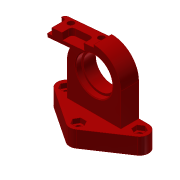
# Autodesk Inventor part: CyclmarcoTraseroY
Saved by Autodesk Inventor 2015 SP2 (Build 190223200, 223)
## iProperties
Created: 2015-05-19
Material: Genérico
Document SubType Name: Modeling
Designer: E.Beroiz
Density: 1 g/cm^3
Appearance: Suave - Rojo
Description: CyclmarcoTraseroY
Author: EDU
Autodesk Inventor part; units mm, degrees
sketch "Boceto1" plane through (0, 0, 0) normal (0, 0, 1) x (1, 0, 0)
  line L0 (-3.0509, -4.5763) -> (-25.5509, 10.4237)
  arc A0 (-22.5, 20.5) -> (-25.5509, 10.4237) centre (-22.5, 15) ccw
  line L1 (-22.5, 20.5) -> (22.5, 20.5)
  arc A1 (25.5509, 10.4237) -> (22.5, 20.5) centre (22.5, 15) ccw
  line L2 (25.5509, 10.4237) -> (3.0509, -4.5763)
  arc A2 (-3.0509, -4.5763) -> (3.0509, -4.5763) centre (0, 0) ccw
  line L3 (22.5, 15) -> (-22.5, 15) construction
  line L4 (0, 15) -> (0, 0) construction
  dimension "d0" = 45
  dimension "d1" = 5.5
  dimension "d2" = 5.5
  dimension "d3" = 5.5
  dimension "d98" = 15
  constraints: 10 end point, 6 point on circle, 6 tangent, 3 centre point, 3 coincident, 1 horizontal, 1 midpoint, 1 perpendicular
  measures "d0" distance of L3.end L3.start
  measures "d1" radius of A1
  measures "d2" radius of A2
  measures "d3" radius of A0
  measures "d98" distance of L4.start L4.end
extrude "Extrusión1" add sketch "Boceto1" along normal blind 10
hole "Agujero1" at (-22.5, 15, 10) direction (0, 0, -1) diameter 3.75 end through all
hole "Agujero2" at (0, 0, 10) direction (0, 0, -1) diameter 3.75 end through all
hole "Agujero3" at (22.5, 15, 10) direction (0, 0, -1) diameter 3.75 end through all
sketch "Boceto3" plane through (0, 0, 10) normal (0, 0, 1) x (1, 0, 0)
  circle A0 centre (22.5, 15) radius 1.875 projected
  circle A1 centre (0, 0) radius 1.875 projected
  circle A2 centre (-22.5, 15) radius 1.875 projected
  line L0 (-25.5509, 10.4237) -> (-3.0509, -4.5763) projected
  arc A3 (-3.0509, -4.5763) -> (3.0509, -4.5763) centre (0, 0) ccw projected
  line L1 (3.0509, -4.5763) -> (25.5509, 10.4237) projected
  arc A4 (25.5509, 10.4237) -> (22.5, 20.5) centre (22.5, 15) ccw projected
  line L2 (22.5, 20.5) -> (-22.5, 20.5) projected
  arc A5 (-22.5, 20.5) -> (-25.5509, 10.4237) centre (-22.5, 15) ccw projected
  line L3 (-20.7001, 18.1175) -> (-18.9002, 15)
  line L4 (-18.9002, 15) -> (-20.7001, 11.8825)
  line L5 (-20.7001, 11.8825) -> (-24.2999, 11.8825)
  line L6 (-24.2999, 11.8825) -> (-26.0998, 15)
  line L7 (-26.0998, 15) -> (-24.2999, 18.1175)
  line L8 (-24.2999, 18.1175) -> (-20.7001, 18.1175)
  line L9 (1.7999, 3.1175) -> (3.5998, 0)
  line L10 (3.5998, 0) -> (1.7999, -3.1175)
  line L11 (1.7999, -3.1175) -> (-1.7999, -3.1175)
  line L12 (-1.7999, -3.1175) -> (-3.5998, 0)
  line L13 (-3.5998, 0) -> (-1.7999, 3.1175)
  line L14 (-1.7999, 3.1175) -> (1.7999, 3.1175)
  line L15 (25.4952, 16.9968) -> (25.7269, 13.4045)
  line L16 (25.7269, 13.4045) -> (22.7317, 11.4077)
  line L17 (22.7317, 11.4077) -> (19.5048, 13.0032)
  line L18 (19.5048, 13.0032) -> (19.2731, 16.5955)
  line L19 (19.2731, 16.5955) -> (22.2683, 18.5923)
  line L20 (22.2683, 18.5923) -> (25.4952, 16.9968)
  line L21 (22.5, 20.5) -> (-22.5, 20.5) projected
  line L22 (3.0509, -4.5763) -> (25.5509, 10.4237) projected
  point P0 (-22.5, 15)
  dimension "d35" = 6.235
  dimension "d36" = 6.235
  dimension "d37" = 6.235
  constraints: 36 end point, 3 coincident, 2 parallel, 1 horizontal, 39 other
  measures "d35" distance between parallel lines of L5 L8
  measures "d36" distance between parallel lines of L12 L9
  measures "d37" distance between parallel lines of L16 L19
extrude "Extrusión2" cut sketch "Boceto3" against normal blind 2.8 contours L3 L4 L5 L6 L7 L8 | L9 L10 L11 L12 L13 L14 | L15 L16 L17 L18 L19 L20
sketch "Boceto4" plane through (0, 0, 10) normal (0, 0, 1) x (1, 0, 0)
  line L0 (22.2683, 18.5923) -> (25.4952, 16.9968) projected
  line L1 (25.4952, 16.9968) -> (25.7269, 13.4045) projected
  line L2 (25.7269, 13.4045) -> (22.7317, 11.4077) projected
  line L3 (22.7317, 11.4077) -> (19.5048, 13.0032) projected
  line L4 (19.5048, 13.0032) -> (19.2731, 16.5955) projected
  line L5 (19.2731, 16.5955) -> (22.2683, 18.5923) projected
  line L6 (-24.2999, 18.1175) -> (-20.7001, 18.1175) projected
  line L7 (-20.7001, 18.1175) -> (-18.9002, 15) projected
  line L8 (-18.9002, 15) -> (-20.7001, 11.8825) projected
  line L9 (-20.7001, 11.8825) -> (-24.2999, 11.8825) projected
  line L10 (-24.2999, 11.8825) -> (-26.0998, 15) projected
  line L11 (-26.0998, 15) -> (-24.2999, 18.1175) projected
  line L12 (-1.7999, 3.1175) -> (1.7999, 3.1175) projected
  line L13 (1.7999, 3.1175) -> (3.5998, 0) projected
  line L14 (3.5998, 0) -> (1.7999, -3.1175) projected
  line L15 (1.7999, -3.1175) -> (-1.7999, -3.1175) projected
  line L16 (-1.7999, -3.1175) -> (-3.5998, 0) projected
  line L17 (-3.5998, 0) -> (-1.7999, 3.1175) projected
  line L18 (-25.5509, 10.4237) -> (-3.0509, -4.5763) projected
  arc A0 (-3.0509, -4.5763) -> (3.0509, -4.5763) centre (0, 0) ccw projected
  line L19 (3.0509, -4.5763) -> (25.5509, 10.4237) projected
  arc A1 (25.5509, 10.4237) -> (22.5, 20.5) centre (22.5, 15) ccw projected
  line L20 (22.5, 20.5) -> (-22.5, 20.5) projected
  arc A2 (-22.5, 20.5) -> (-25.5509, 10.4237) centre (-22.5, 15) ccw projected
  line L21 (22.5, 20.5) -> (-22.5, 20.5) projected
  line L22 (-16.5, 20.5) -> (-16.5, 9.5)
  line L23 (-16.5, 9.5) -> (16.5, 9.5)
  line L24 (16.5, 9.5) -> (16.5, 20.5)
  dimension "d40" = 33
  dimension "d41" = 11
  dimension "d42" = 6
  dimension "d43" = 6
  constraints: 6 end point, 2 parallel, 2 perpendicular, 2 point on line
  measures "d40" distance of L22.end L23.end
  measures "d41" distance of L22.start L22.end
  measures "d42" distance from line of A2.centre L22
  measures "d43" distance from line of L24 A1.centre
extrude "Extrusión3" add sketch "Boceto4" along normal blind 36.5 contours L20 L24 L23 L22
fillet "Empalme1" radius 16.5 2 edges at (-16.5, 15, 46.5) (16.5, 15, 46.5)
hole "Agujero4" at (0, 9.5, 30) direction (0, 1, 0) diameter 22.5 end through all
sketch "Boceto5" plane through (-16.5, 9.5, 10) normal (0, -1, 0) x (1, 0, 0)
  line L0 (1.8522, 27.5956) -> (-11.8667, 26.3953)
  line L1 (-11.8667, 26.3953) -> (-12.3896, 32.3725)
  line L2 (-12.3896, 32.3725) -> (16.5, 34.9)
  line L3 (-9.0509, 0) -> (13.4491, 0) projected
  arc A0 (33, 20) -> (0, 20) centre (16.5, 20) ccw projected
  arc A1 (16.5, 34.9) -> (1.8522, 27.5956) centre (18.4458, 12.6589) ccw
  point P0 (16.5, -10)
  dimension "d56" = 5
  dimension "d57" = 6
  dimension "d58" = 29
  dimension "d59" = 14.9
  constraints: 6 end point, 3 point on circle, 1 centre point, 1 parallel, 1 perpendicular, 1 tangent, 1 vertical alignment
  measures "d56" angle of L3 L0
  measures "d57" distance of L0.end L1.end
  measures "d58" distance of L1.end L2.end
  measures "d59" distance of A0.centre L2.end
extrude "Extrusión4" add sketch "Boceto5" against normal blind 11
sketch "Boceto6" plane through (-16.5, 9.5, 10) normal (0, -1, 0) x (1, 0, 0)
  line L0 (-12.3896, 32.3725) -> (8.0277, 34.1588) projected
  line L1 (8.0277, 34.1588) -> (16.5, 34.9)
  line L2 (-12.3896, 32.3725) -> (8.0277, 34.1588) projected
  line L3 (19.5509, 0) -> (13.4491, 0) projected
  line L4 (16.5, 34.9) -> (16.2385, 37.8886)
  line L5 (16.2385, 37.8886) -> (-12.3896, 32.3725)
  point P0 (16.5, -10)
  point P1 (16.5, 0)
  dimension "d64" = 3
  dimension "d67" = 90
  constraints: 6 end point, 1 collinear, 1 midpoint, 1 vertical alignment
  measures "d64" distance of L1.end L4.end
  measures "d67" angle of L1 L4
extrude "Extrusión5" cut sketch "Boceto6" against normal blind 11
sketch "Boceto7" plane through (22.5, 20.5, 10) normal (0, 1, 0) x (1, 0, 0)
  circle A0 centre (-22.5, -20) radius 11.25 projected
  circle A1 centre (-22.5, -20) radius 10
  point P0 (-22.5, 10)
  dimension "d107" = 20
  constraints: 1 centre point, 1 coincident
  measures "d107" diameter of A1
extrude "Extrusión6" add sketch "Boceto7" against normal blind 7.5
sketch "Boceto9" plane through (-28.8896, 9.5, 42.3725) normal (-0.0871557, 0, 0.9961947) x (0.9961947, 0, 0.0871557)
  line L0 (11.2642, 11) -> (11.2642, 0) projected
  line L1 (0, 11) -> (29, 11) projected
  line L2 (0, 0) -> (0, 11) projected
  line L3 (29, 0) -> (0, 0) projected
  line L4 (29, 0) -> (29, 11) projected
  line L5 (0, 9) -> (1, 9)
  line L6 (3, 7) -> (3, 0)
  line L7 (3, 0) -> (0, 0)
  line L8 (0, 0) -> (0, 9)
  line L9 (11.25, 6) -> (20.75, 6)
  line L10 (22.75, 4) -> (22.75, 0)
  line L11 (22.75, 0) -> (9.25, 0)
  line L12 (9.25, 0) -> (9.25, 4)
  arc A0 (11.25, 6) -> (9.25, 4) centre (11.25, 4) ccw
  arc A1 (22.75, 4) -> (20.75, 6) centre (20.75, 4) ccw
  arc A2 (3, 7) -> (1, 9) centre (1, 7) ccw
  point P0 (25.0867, -9.5)
  point P1 (3, 9)
  point P2 (9.25, 6)
  point P3 (22.75, 6)
  dimension "d81" = 3
  dimension "d82" = 9
  dimension "d83" = 6
  dimension "d86" = 13.5
  dimension "d117" = 9.25
  dimension "d118" = 2
  dimension "d119" = 2
  constraints: 16 end point, 8 point on line, 6 point on circle, 6 tangent, 4 parallel, 3 centre point, 2 horizontal, 2 perpendicular, 1 equal radius, 1 horizontal alignment
  measures "d81" distance of L6.end L7.end
  measures "d82" distance of point (3, 9) L6.end
  measures "d83" distance of point (22.75, 6) L10.end
  measures "d86" distance of point (9.25, 6) point (22.75, 6)
  measures "d117" distance between parallel lines of L12 L8
  measures "d118" radius of A0
  measures "d119" radius of A2
extrude "Extrusión8" cut sketch "Boceto9" against normal blind 4 contours L9 A1 L10 L3 L0 | L0 L3 L12 A0 L9 | L5 A2 L6 L3 L2
fillet "Empalme2" radius 2 1 edges at (-28.6282, 20.5, 39.3839)
sketch "Boceto8" plane through (-28.8896, 9.5, 42.3725) normal (-0.0871557, 0, 0.9961947) x (0.9961947, 0, 0.0871557)
  circle A0 centre (6.75, 8) radius 1.875
  circle A1 centre (25.5, 8) radius 1.875
  line L0 (25.5, 8) -> (6.75, 8) construction
  line L1 (2, 11) -> (29, 11) projected
  line L2 (0, 0) -> (0, 9) projected
  point P0 (25.0867, -9.5)
  dimension "d103" = 3.75
  dimension "d104" = 3.75
  dimension "d108" = 3
  dimension "d109" = 18.75
  dimension "d111" = 6.75
  constraints: 2 centre point, 2 end point, 1 horizontal
  measures "d103" diameter of A0
  measures "d104" diameter of A1
  measures "d108" distance between parallel lines of L0 L1
  measures "d109" distance of L0.start L0.end
  measures "d111" distance from line of L2 L0.end
ref_plane "Plano de trabajo1" through (0.2179, 9.5, 42.4095) normal (-0.0871557, 0, 0.9961947) x (0.9961947, 0, 0.0871557)
extrude "Extrusion11" cut sketch "Boceto8" against normal blind 10
sketch "Boceto10" plane through (0.2179, 9.5, 42.4095) normal (-0.0871557, 0, 0.9961947) x (0.9961947, 0, 0.0871557)
  line L0 (-25.3675, 6.2001) -> (-25.3675, 9.7999)
  line L1 (-19.1325, 9.7999) -> (-19.1325, 6.2001)
  line L2 (-19.1325, 6.2001) -> (-22.25, 4.4002)
  line L3 (-22.25, 4.4002) -> (-25.3675, 6.2001)
  line L4 (-0.3825, 9.796) -> (-0.3825, 6.2001)
  line L5 (-0.3825, 6.2001) -> (-3.5, 4.4002)
  line L6 (-3.5, 4.4002) -> (-6.6175, 6.2001)
  line L7 (-6.6175, 6.2001) -> (-6.6175, 9.8038)
  line L8 (-25.3675, 9.7999) -> (-25.3675, 12.5)
  line L9 (-25.3675, 12.5) -> (-19.1325, 12.5)
  line L10 (-19.1325, 12.5) -> (-19.1325, 9.7999)
  line L11 (-6.6175, 9.8038) -> (-6.6175, 12)
  line L12 (-6.6175, 12) -> (-0.3825, 12)
  line L13 (-0.3825, 12) -> (-0.3825, 9.796)
  line L14 (-27, 11) -> (0, 11) projected
  circle A0 centre (-22.25, 8) radius 1.875 projected
  circle A1 centre (-3.5, 8) radius 3.1175 construction
  circle A2 centre (-3.5, 8) radius 1.875 projected
  point P0 (-3.9133, -9.5)
  point P1 (-1.625, 8)
  point P2 (-14.4848, 20.8557)
  dimension "d91" = 6.235
  dimension "d92" = 6.235
  dimension "d114" = 1.5
  dimension "d115" = 1
  dimension "d116" = 120
  constraints: 28 end point, 4 perpendicular, 4 tangent, 4 vertical, 2 coincident, 1 centre point, 1 horizontal alignment, 1 vertical alignment, 8 other
  measures "d91" distance between parallel lines of L1 L0
  measures "d92" distance between parallel lines of L4 L7
  measures "d114" distance between parallel lines of L14 L9
  measures "d115" distance between parallel lines of L12 L14
  measures "d116" angle of L5 L6
extrude "Extrusión9" cut sketch "Boceto10" against normal blind 4 contours L0 L8 L14 L10 L1 L2 L3 | L8 L9 L10 L14 | L4 L5 L6 L7 L11 L14 L13 | L14 L11 L12 L13 | A0 | A2
chamfer "Chaflán3" distance 0.5 angle 30 1 edges at (0, 9.5, 41.25) measured on face at (0, 9.5, 12.9167)
